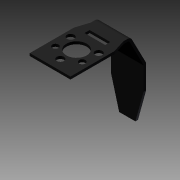
# Autodesk Inventor part: ASAP_Top_Fixture_New
Saved by Autodesk Inventor 2011 SP2 (Build 150309200, 309)
## iProperties
Created: 2011-11-18
Part Number: ASAP_Top_Fixture_New
Material: Default
Document SubType Name: Sheet Metal
Designer: sungwook
Density: 1 g/cm^3
Sheet Metal Rule: Default_mm
Flat Pattern Width: 1 cm
Flat Pattern Length: 3.65103 cm
Flat Pattern Area: 3.65103 cm^2
Sheet Metal Width: 10.000 mm
Sheet Metal Length: 36.510 mm
Sheet Metal Area: 365.103 mm^2
Author: sungwook
Autodesk Inventor part; units mm, degrees
ref_plane "YZ Plane" through (0, 0, 0) normal (1, 0, 0) x (0, 1, 0)
ref_plane "XZ Plane" through (0, 0, 0) normal (0, 1, 0) x (-1, 0, 0)
ref_plane "XY Plane" through (0, 0, 0) normal (0, 0, 1) x (1, 0, 0)
sketch "Sketch1" plane through (0, 0, 0) normal (0, 0, 1) x (1, 0, 0)
  line L0 (0, -10.3907) -> (0, 16.8443)
  line L1 (-4, 7.5) -> (4, 7.5)
  line L2 (4, 7.5) -> (4, 2.1599)
  line L3 (4, 2.1599) -> (-4, 2.1599)
  line L4 (-4, 2.1599) -> (-4, 7.5)
  line L5 (-7, 0) -> (7, 0)
  line L6 (-4, 7.5) -> (-5, 4.34)
  line L7 (4, 7.5) -> (5, 4.34)
  line L8 (-4, 4.34) -> (4, 4.34)
  line L9 (-5, -6.5) -> (-5, 4.34)
  line L10 (5, 4.34) -> (5, -6.5)
  line L11 (5, -6.5) -> (-5, -6.5)
  line L12 (-4, 7.5) -> (4, 7.5)
  line L13 (4, 7.5) -> (4, 8.5)
  line L14 (4, 8.5) -> (-4, 8.5)
  line L15 (-4, 8.5) -> (-4, 7.5)
  point P0 (0, 7.5)
  point P1 (0, 0)
  dimension "d6" = 8
  dimension "d9" = 10.84
  dimension "d40" = 7.5
  dimension "d41" = 8.5
extrude "Plate1" add sketch "Sketch1" along normal blind 0.635
sketch "Sketch2" plane through (0, 0, 0.635) normal (0, 0, 1) x (1, 0, 0)
  circle A0 centre (0, 0) radius 2.5019
  line L0 (0, -10.3907) -> (0, 16.8443) projected
  point P0 (0, -3.9878)
  dimension "d12" = 5.0038
  dimension "d69" = 3.9878
  constraints: 1 centre point, 1 coincident, 1 point on line
  measures "d12" diameter of A0
  measures "d69" distance of point (0, -3.988) point (0, 0)
extrude "Cut1" cut sketch "Sketch2" against normal blind 0.635
hole "Hole1" at (0, -3.9878, 0.635) direction (0, 0, -1) diameter 1.778 end through all
pattern_circular "Circular Pattern1" count 3 over 360 about axis through (0, 0, -10) along (0, 0, 1) of "Hole1"
sketch "Sketch3" plane through (0, 0, 0.635) normal (0, 0, 1) x (1, 0, 0)
  circle A0 centre (0, 0) radius 2.5019 projected
  line L0 (-2.5, 5.334) -> (2.5, 5.334)
  line L1 (2.5, 5.334) -> (2.5, 4.572)
  line L2 (2.5, 4.572) -> (-2.5, 4.572)
  line L3 (-2.5, 4.572) -> (-2.5, 5.334)
  point P0 (0, 5.334)
  dimension "d25" = 5
  dimension "d26" = 0.762
  dimension "d27" = 5.334
  constraints: 8 end point, 2 parallel, 1 horizontal, 1 midpoint, 1 perpendicular, 1 vertical alignment
  measures "d25" distance of L0.end L0.start
  measures "d26" distance between parallel lines of L2 L0
  measures "d27" distance from line of A0.centre L0
cut "Cut2" [suppressed]
sketch "Sketch5" plane through (4, 9.0633, -0.3418) normal (0, 0.8870108, 0.4617486) x (-1, 0, 0)
  line L0 (8, 0) -> (0, 0)
  line L1 (0, 0) -> (0, -7.2293)
  line L2 (0, -7.2293) -> (8, -7.2293)
  line L3 (8, -7.2293) -> (8, 0)
  constraints: 4 end point, 4 other
edge flange "Flange2" height 8 angle 62.5 thickness 0.635 bend radius 0.635 thickness toward (0, 0.8870108, 0.4617486) relief straight relief width 0.635 relief depth 0.3175 edges at (0, 8.5, 0) wall of the first edge with corners at (-4, 9.0633, -0.3418) (4, 9.0633, -0.3418) (4, 12.4014, -6.7543) (-4, 12.4014, -6.7543)
bend "Bend2"
corner "Corner2"
sketch "Sketch6" plane through (-4, 12.4731, -7.0475) normal (0, 1, 0) x (1, 0, 0)
  line L0 (8, 0) -> (0, 0)
  line L1 (0, 0) -> (0, -12.8446)
  line L2 (0, -12.8446) -> (8, -12.8446)
  line L3 (8, -12.8446) -> (8, 0)
  constraints: 4 end point, 4 other
edge flange "Flange3" height 13 angle -27.5 thickness 0.635 bend radius 0.635 thickness toward (0, 1, 0) relief straight relief width 0.635 relief depth 0.3175 edges at (0, 12.9646, -6.4611) wall of the first edge with corners at (4, 12.4731, -7.0475) (-4, 12.4731, -7.0475) (-4, 12.4731, -19.8921) (4, 12.4731, -19.8921)
bend "Bend3"
corner "Corner3"
sketch "Sketch8" plane through (-4, 13.1081, -19.8921) normal (0, 1, 0) x (1, 0, 0)
  line L0 (0, -12.8446) -> (8, -12.8446) projected
  line L1 (8, -12.8446) -> (8, 0) projected
  line L2 (8, 0) -> (0, 0) projected
  line L3 (0, -12.8446) -> (0, 0) projected
  line L4 (2, 0) -> (6, 0)
  line L5 (6, 0) -> (6, -10.36)
  line L6 (6, -10.36) -> (2, -10.36)
  line L7 (2, -10.36) -> (2, 0)
  line L8 (4, 4.1054) -> (4, -24.6325) projected
  line L9 (2, 0) -> (0, -7.32)
  line L10 (6, 0) -> (8, -7.32)
  line L11 (0, -7.32) -> (0, 0)
  line L12 (2, 0) -> (0, 0)
  line L13 (6, 0) -> (8, 0)
  line L14 (8, -7.32) -> (8, 0)
  point P0 (4, -19.8921)
  point P1 (4, 0)
  point P2 (4, 0)
  dimension "d63" = 4
  dimension "d64" = 7.32
  dimension "d65" = 12.8446
  constraints: 20 end point, 4 collinear, 2 midpoint, 2 parallel, 2 point on line, 1 coincident, 1 horizontal, 1 perpendicular, 1 symmetric about line
  measures "d63" distance between parallel lines of L5 L7
  measures "d64" vertical distance of L4.start L9.end
  measures "d65" distance between parallel lines of L0 L2
extrude "Cut3" cut sketch "Sketch8" against normal blind 0.635 contours L3 L2 L9 | L10 L2 L1
sketch "Sketch9" plane through (5, -6.5, 0) normal (1, 0, 0) x (0, 0, -1)
  line L0 (-0.635, 10.84) -> (-0.635, 0) projected
  line L1 (0, 0) -> (-0.635, 0) projected
  line L2 (0, 0) -> (0, 10.84) projected
  line L3 (0, 10.84) -> (-0.635, 10.84) projected
  line L4 (0.0486, 16.1265) -> (0.3418, 15.5633) projected
  arc A0 (0.0486, 16.1265) -> (-0.635, 15) centre (0.635, 15) ccw projected
  line L5 (0, 15) -> (-0.635, 15) projected
  arc A1 (0.3418, 15.5633) -> (0, 15) centre (0.635, 15) ccw projected
  line L6 (0, 14) -> (0, 15) projected
  line L7 (7.0475, 19.6081) -> (7.0475, 18.9731) projected
  arc A2 (7.0475, 19.6081) -> (6.4611, 19.4646) centre (7.0475, 18.3381) ccw projected
  line L8 (6.7543, 18.9014) -> (6.4611, 19.4646) projected
  arc A3 (7.0475, 18.9731) -> (6.7543, 18.9014) centre (7.0475, 18.3381) ccw projected
  line L9 (-0.635, 15) -> (15.1902, 15)
  line L10 (0.0486, 16.1265) -> (6.4611, 19.4646)
  point P0 (0, 6.5)
  constraints: 4 end point, 2 perpendicular, 1 tangent
sketch "Sketch10" plane through (0, 0, 0.635) normal (0, 0, 1) x (1, 0, 0)
  circle A0 centre (0, 0) radius 2.5019 projected
  line L0 (-2.54, 5.7658) -> (2.54, 5.7658)
  line L1 (2.54, 5.7658) -> (2.54, 4.4958)
  line L2 (2.54, 4.4958) -> (-2.54, 4.4958)
  line L3 (-2.54, 4.4958) -> (-2.54, 5.7658)
  point P0 (0, 5.7658)
  dimension "d70" = 1.27
  dimension "d71" = 5.08
  dimension "d72" = 4.4958
  constraints: 8 end point, 2 parallel, 1 horizontal, 1 midpoint, 1 perpendicular, 1 vertical alignment
  measures "d70" distance between parallel lines of L2 L0
  measures "d71" distance of L0.end L0.start
  measures "d72" distance from line of A0.centre L2
extrude "Cut4" cut sketch "Sketch10" against normal blind 0.635 contours L0 L1 L2 L3
sketch "Sketch11" plane through (0, 0, 0.635) normal (0, 0, 1) x (1, 0, 0)
  circle A0 centre (0, 0) radius 2.5019 projected
  line L0 (0, -10.4287) -> (0, 17.0722) projected
  circle A1 centre (-3.2996, -1.905) radius 0.762
  circle A2 centre (3.2996, -1.905) radius 0.762
  point P0 (0, 3.81)
  point P1 (3.2996, -1.905)
  dimension "d75" = 3.81
  dimension "d78" = 360
  dimension "d80" = 1.524
  constraints: 2 centre point, 1 coincident, 1 symmetric about line, 5 other
  measures "d75" distance of A0.centre point (0, 3.81)
  measures "d80" diameter of A1
extrude "Cut5" cut sketch "Sketch11" against normal blind 0.635 contours A1 | A2
equation "\"d13\" = Thickness"
equation "\"d20\" = Thickness"
equation "\"d28\" = Thickness"
equation "\"d66\" = Thickness"
equation "\"d73\" = Thickness"
equation "\"d81\" = Thickness"
equation "\"d42\" = BendReliefWidth"
equation "\"d43\" = BendReliefDepth"
equation "\"d44\" = MinimumRemnant"
equation "\"d45\" = BendRadius"
equation "\"d48\" = BendRadius"
equation "\"d49\" = CornerReliefSize"
equation "\"d50\" = GapSize"
equation "\"d51\" = JacobiRadiusSize"
equation "\"d52\" = BendReliefWidth"
equation "\"d53\" = BendReliefDepth"
equation "\"d54\" = MinimumRemnant"
equation "\"d55\" = BendRadius"
equation "\"d58\" = BendRadius"
equation "\"d59\" = CornerReliefSize"
equation "\"d60\" = GapSize"
equation "\"d61\" = JacobiRadiusSize"
equation "\"BendRadius\" = Thickness"
equation "\"BendReliefWidth\" = Thickness"
equation "\"BendReliefDepth\" = 0.5 * Thickness"
equation "\"CornerReliefSize\" = 4 * Thickness"
equation "\"MinimumRemnant\" = 2 * Thickness"
equation "\"TransitionRadius\" = BendRadius"
equation "\"JacobiRadiusSize\" = BendRadius"
equation "\"GapSize\" = Thickness"
equation "\"d10\" = BendRadius"
equation "\"Thickness\" = 0.635"
body "Solid1"
